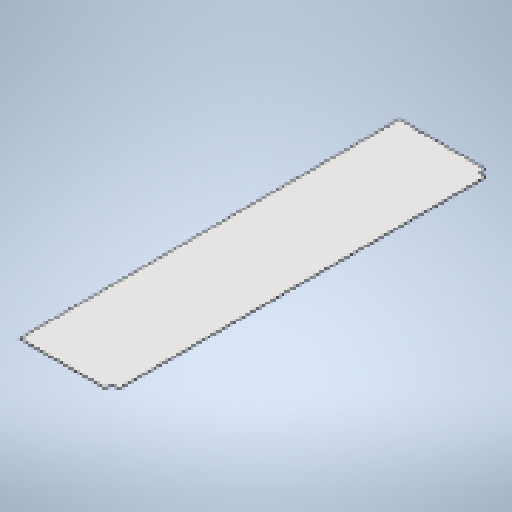
# Autodesk Inventor part: GnG frame 2 floor sheet 10
Saved by Autodesk Inventor 2025.3 (Build 293356000, 356)
## iProperties
Created: 2025-10-28
Part Number: GnG frame 2 floor sheet 10
Material: Stainless Steel
Document SubType Name: Sheet Metal
Designer: admin
Mass: 280.619 g
Surface Area: 364.406 cm^2
Volume: 35.0774 cm^3
Density: 8 g/cm^3
Sheet Metal Rule: AISI304 3mm Die 32
Sheet Metal Width: 0,000 mm
Sheet Metal Length: 0,000 mm
Sheet Metal Area: 0,000 mm^2
Appearance: Default
Author: admin
Autodesk Inventor part; units mm, degrees
ref_plane "YZ Plane" through (0, 0, 0) normal (1, 0, 0) x (0, 1, 0)
ref_plane "XZ Plane" through (0, 0, 0) normal (0, 1, 0) x (-1, 0, 0)
ref_plane "XY Plane" through (0, 0, 0) normal (0, 0, 1) x (1, 0, 0)
sketch "Sketch1" plane through (0, 0, 0) normal (0, 0, 1) x (1, 0, 0)
  line L0 (0, 0) -> (-515, 0)
  line L1 (-515, 0) -> (-515, -2100)
  line L2 (-515, -2100) -> (0, -2100)
  line L3 (0, -2100) -> (0, 0)
  line L4 (0, 0) -> (-40, 0)
  line L5 (-40, 0) -> (-40, -35)
  line L6 (-40, -35) -> (0, -35)
  line L7 (0, -35) -> (0, 0)
  line L8 (0, -2100) -> (-40, -2100)
  line L9 (-40, -2100) -> (-40, -2065)
  line L10 (-40, -2065) -> (0, -2065)
  line L11 (0, -2065) -> (0, -2100)
  line L12 (-515, 0) -> (-475, 0)
  line L13 (-475, 0) -> (-475, -35)
  line L14 (-475, -35) -> (-515, -35)
  line L15 (-515, -35) -> (-515, 0)
  line L16 (-515, -2100) -> (-475, -2100)
  line L17 (-475, -2100) -> (-475, -2065)
  line L18 (-475, -2065) -> (-515, -2065)
  line L19 (-515, -2065) -> (-515, -2100)
  line L20 (-340, -2100) -> (-240, -2100)
  line L21 (-240, -2100) -> (-240, -2065)
  line L22 (-240, -2065) -> (-340, -2065)
  line L23 (-340, -2065) -> (-340, -2100)
  line L24 (-340, 0) -> (-240, 0)
  line L25 (-240, 0) -> (-240, -35)
  line L26 (-240, -35) -> (-340, -35)
  line L27 (-340, -35) -> (-340, 0)
  point P0 (0, -35)
  point P1 (-40, 0)
  point P2 (-40, -2100)
  point P3 (0, -2065)
  point P4 (-240, 0)
  point P5 (-475, 0)
  point P6 (-515, -35)
  point P7 (-515, -2065)
  point P8 (-515, -35)
  point P9 (-515, -2065)
  dimension "d22" = 515
  dimension "d23" = 2100
  dimension "d24" = 40
  dimension "d25" = 35
  dimension "d28" = 100
  dimension "d29" = 200
  measures "d22" distance of L2.end L1.end
  measures "d23" distance of L1.end L0.end
  measures "d24" distance of L6.end L5.end
  measures "d25" distance of L5.end L4.end
  measures "d28" distance of L25.end L26.end
  measures "d29" distance between parallel lines of L5 L25
extrude "Plate1" add sketch "Sketch1" along normal blind 3 contours L5 L6 L3 L10 L9 L2 L21 L22 L23 L17 L18 L1 L14 L13 L0 L27 L26 L25 | L25 L26 L27 L0 | L13 L14 L1 L0 | L2 L23 L22 L21 | L18 L17 L2 L1
sketch "Sketch5" plane through (0, 0, 0) normal (0, 0, -1) x (-1, 0, 0)
  line L0 (515, 0) -> (415, 0) construction
  line L1 (415, 0) -> (415, -2) construction
  line L2 (415, -2) -> (515, -2) construction
  line L3 (515, -2) -> (515, 0) construction
  line L4 (415, 0) -> (413.4752, -4.6556)
  arc A0 (412.5248, -4.6556) -> (413.4752, -4.6556) centre (413, -4.5) ccw
  line L5 (412.5248, -4.6556) -> (411, 0)
  line L6 (411, 0) -> (415, 0)
  line L7 (411, 0) -> (409, 0) construction
  line L8 (409, 0) -> (407, 0)
  line L9 (407, 0) -> (407, -5)
  line L10 (407, -5) -> (409, -5)
  line L11 (409, -5) -> (409, 0)
  line L12 (407, 0) -> (405, 0) construction
  line L13 (405, 0) -> (403, 0)
  line L14 (403, 0) -> (403, -5)
  line L15 (403, -5) -> (405, -5)
  line L16 (405, -5) -> (405, 0)
  line L17 (403, 0) -> (401, 0) construction
  line L18 (401, 0) -> (399, 0)
  line L19 (399, 0) -> (399, -5)
  line L20 (399, -5) -> (401, -5)
  line L21 (401, -5) -> (401, 0)
  line L22 (399, 0) -> (397, 0) construction
  line L23 (397, 0) -> (395, 0)
  line L24 (395, 0) -> (395, -5)
  line L25 (395, -5) -> (397, -5)
  line L26 (397, -5) -> (397, 0)
  line L27 (395, 0) -> (390, 0) construction
  line L28 (390, 0) -> (385, 0) construction
  circle A1 centre (390, 0) radius 1
  circle A2 centre (385, 0) radius 1
  point P0 (0, 0)
  point P1 (413, 0)
  point P2 (515, 0)
  dimension "d30" = 100
  dimension "d31" = 2
  dimension "d32" = 5
  dimension "d33" = 4
  dimension "d34" = 0.5
  dimension "d35" = 5
  dimension "d36" = 5
  dimension "d37" = 5
  dimension "d38" = 2
  constraints: 58 end point, 11 horizontal, 10 equal length, 10 parallel, 5 perpendicular, 4 coincident, 3 centre point, 3 tangent, 2 point on circle, 1 equal radius, 1 midpoint, 1 point on line, 1 vertical alignment
  measures "d30" distance of L2.end L1.end
  measures "d31" distance of L1.end L0.end
  measures "d32" distance of L9.end L9.start
  measures "d33" distance of L5.end L0.end
  measures "d34" radius of A0
  measures "d35" distance of L15.start L13.end
  measures "d36" distance of L19.end L19.start
  measures "d37" distance of L24.end L24.start
  measures "d38" diameter of A1
extrude "Cut1" cut sketch "Sketch5" against normal blind 3 contours L26 L25 L24 L23 | A1 | A2
equation "\"d33\" = 2 * d31"
equation "\"d34\" = 0.25 * d31"
equation "\"d38\" = d31"
equation "\"d39\" = Thickness"
equation "\"d2\" = Thickness"
equation "\"BendReliefWidth\" = Thickness"
equation "\"BendReliefDepth\" = 0.5 * Thickness"
equation "\"CornerReliefSize\" = 4 * Thickness"
equation "\"MinimumRemnant\" = 2 * Thickness"
equation "\"TransitionRadius\" = BendRadius"
equation "\"JacobiRadiusSize\" = BendRadius"
equation "\"GapSize\" = Thickness"
equation "\"Thickness\" = 3"
equation "\"BendRadius\" = 5"
body "Solid1"
